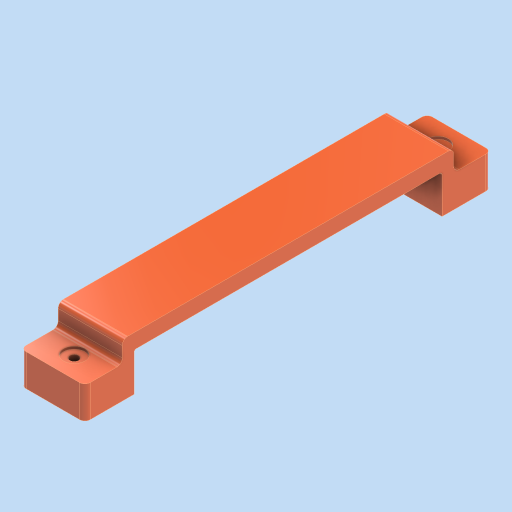
# Autodesk Inventor part: Battery Strap
Saved by Autodesk Inventor 2023 (Build 270158000, 158)
## iProperties
Created: 2023-11-10
Part Number: Battery Strap
Material: Generic
Document SubType Name: Modeling
Designer: adamarnold
Density: 1 g/cm^3
Appearance: Smooth - Light Orange
Mass: 67.6054 g
Surface Area: 258.8 cm^2
Volume: 67.6054 cm^3
Author: adamarnold
Autodesk Inventor part; units mm, degrees
ref_plane "YZ Plane" through (0, 0, 0) normal (1, 0, 0) x (0, 1, 0)
ref_plane "XZ Plane" through (0, 0, 0) normal (0, 1, 0) x (-1, 0, 0)
ref_plane "XY Plane" through (0, 0, 0) normal (0, 0, 1) x (1, 0, 0)
sketch "Sketch1" plane through (0, 0, 0) normal (0, 1, 0) x (-1, 0, 0)
  line L0 (0, 0) -> (38.1, 0)
  line L1 (38.1, 0) -> (38.1, -241.3)
  line L2 (38.1, -241.3) -> (0, -241.3)
  line L3 (0, -241.3) -> (0, 0)
  dimension "d0" = 38.1
  dimension "d1" = 241.3
  constraints: 8 end point, 2 parallel, 1 horizontal, 1 perpendicular
  measures "d0" distance of L1.end L2.end
  measures "d1" distance of L0.end L1.end
extrude "Extrusion1" add sketch "Sketch1" along normal blind 31.75
sketch "Sketch2" plane through (0, 0, 0) normal (1, 0, 0) x (0, 0, -1)
  line L0 (241.3, 0) -> (0, 0) projected
  line L1 (120.65, 0) -> (120.65, 22.86)
  line L2 (120.65, 22.86) -> (212.09, 22.86)
  line L3 (241.3, 31.75) -> (0, 31.75) projected
  line L4 (120.65, 22.86) -> (29.21, 22.86)
  line L5 (29.21, 22.86) -> (29.21, 0)
  line L6 (212.09, 22.86) -> (212.09, 0)
  line L7 (212.09, 0) -> (29.21, 0)
  dimension "d4" = 22.86
  dimension "d5" = 91.44
  dimension "d7" = 91.44
  constraints: 12 end point, 3 perpendicular, 2 point on line, 1 collinear, 1 horizontal, 1 midpoint, 1 vertical
  measures "d4" distance of L1.start L1.end
  measures "d5" distance of L1.end L2.end
  measures "d7" distance of L1.end L4.end
extrude "Extrusion2" cut sketch "Sketch2" against normal through all
fillet "Fillet1" radius 1.27 2 edges at (-19.05, 22.86, -212.09) (-19.05, 22.86, -29.21)
sketch "Sketch5" plane through (0, 0, -241.3) normal (1, 0, 0) x (0, 0, -1)
  line L0 (0, 31.75) -> (-22.225, 31.75)
  line L1 (-22.225, 31.75) -> (-22.225, 19.05)
  line L2 (-22.225, 19.05) -> (0, 19.05)
  line L3 (0, 19.05) -> (0, 31.75)
  line L4 (-241.3, 0) -> (-241.3, 31.75) projected
  line L5 (-241.3, 31.75) -> (-219.075, 31.75)
  line L6 (-219.075, 31.75) -> (-219.075, 19.05)
  line L7 (-219.075, 19.05) -> (-241.3, 19.05)
  line L8 (-241.3, 19.05) -> (-241.3, 31.75)
  dimension "d29" = 22.225
  dimension "d30" = 12.7
  dimension "d31" = 22.225
  dimension "d32" = 12.7
  constraints: 16 end point, 4 parallel, 2 horizontal, 2 perpendicular
  measures "d29" distance of L2.end L1.end
  measures "d30" distance of L1.end L0.end
  measures "d31" distance of L6.end L7.end
  measures "d32" distance of L5.end L6.end
extrude "Extrusion3" cut sketch "Sketch5" against normal through all
fillet "Fillet2" radius 3.175 4 edges at (-19.05, 19.05, -219.075) (-19.05, 31.75, -219.075) (-19.05, 31.75, -22.225) (-19.05, 19.05, -22.225)
sketch "Sketch6" plane through (-38.1, 19.05, -241.3) normal (0, 1, 0) x (1, 0, 0)
  line L0 (0, 0) -> (38.1, 0) projected
  line L1 (38.1, 0) -> (38.1, -19.05) projected
  point P0 (38.1, -241.3)
  point P1 (19.05, -12.7)
  dimension "d36" = 12.7
  dimension "d44" = 19.05
  measures "d36" distance from line of L0 point (19.05, -12.7)
  measures "d44" distance from line of L1 point (19.05, -12.7)
hole "Hole3" at (-19.05, 19.05, -228.6) direction (0, -1, 0) diameter 5.1594 end through all counterbore diameter 12.7 counterbore depth 1.5875
sketch "Sketch7" plane through (-38.1, 19.05, 0) normal (0, 1, 0) x (1, 0, 0)
  line L0 (38.1, 0) -> (0, 0) projected
  line L1 (38.1, 19.05) -> (38.1, 0) projected
  point P0 (19.05, 12.7)
  dimension "d45" = 12.7
  dimension "d46" = 19.05
  measures "d45" distance from line of L0 point (19.05, 12.7)
  measures "d46" distance from line of L1 point (19.05, 12.7)
hole "Hole4" at (-19.05, 19.05, -12.7) direction (0, -1, 0) diameter 5.1594 end through all counterbore diameter 12.7 counterbore depth 1.5875
fillet "Fillet3" radius 3.175 4 edges at (0, 9.525, 0) (-38.1, 9.525, 0) (0, 9.525, -241.3) (-38.1, 9.525, -241.3)
sketch "Sketch11" plane through (0, 0, 0) normal (0, -1, 0) x (1, 0, 0)
  circle A0 centre (-19.05, -228.6) radius 2.5797 projected
  point P0 (0, 0)
  constraints: 1 coincident
hole "Hole5" at (-19.05, 0, -228.6) direction (0, 1, 0) diameter 11.43 depth 6.35 tip angle 118
sketch "Sketch12" plane through (0, 0, 0) normal (0, -1, 0) x (1, 0, 0)
  circle A0 centre (-19.05, -12.7) radius 2.5797 projected
  point P0 (0, 0)
  constraints: 1 coincident
hole "Hole6" at (-19.05, 0, -12.7) direction (0, 1, 0) diameter 11.43 depth 6.35 tip angle 118
body "Solid1"
